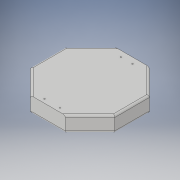
# Autodesk Inventor part: stand_bottom
Saved by Autodesk Inventor 2019 (Build 230136000, 136)
## iProperties
Created: 2019-12-27
Part Number: stand_bottom
Material: Типовые
Document SubType Name: Modeling
Designer: stepa
Density: 1 g/cm^3
Appearance: По умолчанию
Author: stepa
Autodesk Inventor part; units mm, degrees
ref_plane "YZ Plane" through (0, 0, 0) normal (1, 0, 0) x (0, 1, 0)
ref_plane "XZ Plane" through (0, 0, 0) normal (0, 1, 0) x (-1, 0, 0)
ref_plane "XY Plane" through (0, 0, 0) normal (0, 0, 1) x (1, 0, 0)
sketch "Эскиз1" plane through (0, 0, 0) normal (0, 1, 0) x (-1, 0, 0)
  line L0 (108.6396, 45) -> (108.6396, -45)
  line L1 (108.6396, -45) -> (45, -108.6396)
  line L2 (45, -108.6396) -> (-45, -108.6396)
  line L3 (-45, -108.6396) -> (-108.6396, -45)
  line L4 (-108.6396, -45) -> (-108.6396, 45)
  line L5 (-108.6396, 45) -> (-45, 108.6396)
  line L6 (-45, 108.6396) -> (45, 108.6396)
  line L7 (45, 108.6396) -> (108.6396, 45)
  point P0 (0, 0)
  point P1 (0, 0)
  dimension "d0" = 90
  constraints: 16 end point, 1 coincident, 1 horizontal, 17 other
  measures "d0" distance of L0.start L0.end
extrude "Выдавливание1" add sketch "Эскиз1" along normal blind 40
sketch "Эскиз2" plane through (0, 40, 0) normal (0, 1, 0) x (1, 0, 0)
  line L0 (-108.6396, 45) -> (-108.6396, -45) projected
  line L1 (-108.6396, -45) -> (-45, -108.6396) projected
  line L2 (-45, -108.6396) -> (45, -108.6396) projected
  line L3 (45, -108.6396) -> (108.6396, -45) projected
  line L4 (108.6396, -45) -> (108.6396, 45) projected
  line L5 (108.6396, 45) -> (45, 108.6396) projected
  line L6 (45, 108.6396) -> (-45, 108.6396) projected
  line L7 (-45, 108.6396) -> (-108.6396, 45) projected
  point P0 (0, 0)
  point P1 (-18.8883, -98.6396)
  point P2 (21.1117, -98.6396)
  point P3 (-13.7506, 93.6396)
  point P4 (16.2494, 93.6396)
  dimension "d3" = 40
  dimension "d4" = 10
  dimension "d12" = 30
  dimension "d13" = 15
  constraints: 2 horizontal alignment
  measures "d3" distance of point (21.112, -98.64) point (-18.888, -98.64)
  measures "d4" distance from line of L2 point (-18.888, -98.64)
  measures "d12" distance of point (16.249, 93.64) point (-13.751, 93.64)
  measures "d13" distance from line of L6 point (-13.751, 93.64)
hole "Отверстие1" at (-18.8883, 40, 98.6396) at (21.1117, 40, 98.6396) at (-13.7506, 40, -93.6396) at (16.2494, 40, -93.6396) direction (0, -1, 0) diameter 3 end through all
fillet "Сопряжение1" radius 5 14 edges at (-76.8198, 40, 76.8198) (-108.6396, 40, 0) (-76.8198, 40, -76.8198) (76.8198, 40, 76.8198) (108.6396, 40, 0) (76.8198, 40, -76.8198) (76.8198, 0, -76.8198) (108.6396, 0, 0) (76.8198, 0, 76.8198) (0, 0, -108.6396) (-76.8198, 0, -76.8198) (-108.6396, 0, 0) (-76.8198, 0, 76.8198) (0, 0, 108.6396)
